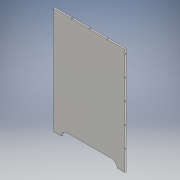
# Autodesk Inventor part: Venstre side mk2
Saved by Autodesk Inventor 2016 (Build 200138000, 138)
## iProperties
Created: 2015-10-17
Part Number: Venstre side mk2
Material: Generic
Document SubType Name: Modeling
Designer: iLyngklip
Density: 1 g/cm^3
Appearance: White
Author: iLyngklip
Autodesk Inventor part; units mm, degrees
ref_plane "YZ Plane" through (0, 0, 0) normal (1, 0, 0) x (0, 1, 0)
ref_plane "XZ Plane" through (0, 0, 0) normal (0, 1, 0) x (-1, 0, 0)
ref_plane "XY Plane" through (0, 0, 0) normal (0, 0, 1) x (1, 0, 0)
sketch "Sketch1" plane through (0, 0, 0) normal (0, 1, 0) x (-1, 0, 0)
  line L0 (160, 240) -> (-160, 240)
  line L1 (-160, 240) -> (-160, -240)
  line L2 (-160, -240) -> (160, -240)
  line L3 (160, -240) -> (160, 240)
  point P0 (0, 0)
  dimension "d0" = 320
  dimension "d1" = 480
  dimension "d2" = 240
  dimension "d3" = 160
  constraints: 8 end point, 2 parallel, 1 horizontal, 1 perpendicular
  measures "d0" distance of L1.end L2.end
  measures "d1" distance of L2.end L0.start
  measures "d2" distance from line of point (0, 0) L0
  measures "d3" distance from line of point (0, 0) L3
extrude "Tykkelse" add sketch "Sketch1" along normal blind 6
sketch "Sketch2" plane through (0, 6, 0) normal (0, 1, 0) x (1, 0, 0)
  line L0 (160, 240) -> (-160, 240) construction
  arc A0 (100, 215) -> (125, 240) centre (100, 240) ccw
  arc A1 (-125, 240) -> (-100, 215) centre (-100, 240) ccw
  line L1 (-100, 215) -> (100, 215)
  line L2 (-125, 240) -> (125, 240)
  point P0 (0, 0)
  dimension "d6" = 50
  dimension "d7" = 50
  dimension "d8" = 60
  dimension "d9" = 60
  constraints: 4 end point, 4 point on circle, 4 point on line, 2 centre point, 1 collinear, 1 horizontal, 1 tangent
  measures "d6" diameter of A0
  measures "d7" diameter of A1
  measures "d8" distance of L0.start A0.centre
  measures "d9" distance of A1.centre L0.end
extrude "Fødder" cut sketch "Sketch2" against normal up to surface (6 mm away)
sketch "Sketch7" plane through (0, 6, 0) normal (0, 1, 0) x (1, 0, 0)
  line L0 (-160, 146.5) -> (-153.679, 146.5) projected
  line L1 (-160, 149.5) -> (-160, 146.5) projected
  line L2 (-153.679, 149.5) -> (-160, 149.5) projected
  arc A0 (-152.2, 150.75) -> (-153.679, 149.5) centre (-152.2, 149.25) ccw projected
  line L3 (-150.8, 150.75) -> (-152.2, 150.75) projected
  arc A1 (-149.302, 149.3277) -> (-150.8, 150.75) centre (-150.8, 149.25) ccw projected
  arc A2 (-149.302, 146.6723) -> (-149.302, 149.3277) centre (-150, 148) ccw projected
  arc A3 (-150.8, 145.25) -> (-149.302, 146.6723) centre (-150.8, 146.75) ccw projected
  line L4 (-152.2, 145.25) -> (-150.8, 145.25) projected
  arc A4 (-153.679, 146.5) -> (-152.2, 145.25) centre (-152.2, 146.75) ccw projected
  line L5 (-150.8, 58.75) -> (-152.2, 58.75) projected
  arc A5 (-149.302, 57.3277) -> (-150.8, 58.75) centre (-150.8, 57.25) ccw projected
  arc A6 (-149.302, 54.6723) -> (-149.302, 57.3277) centre (-150, 56) ccw projected
  arc A7 (-150.8, 53.25) -> (-149.302, 54.6723) centre (-150.8, 54.75) ccw projected
  line L6 (-152.2, 53.25) -> (-150.8, 53.25) projected
  arc A8 (-153.679, 54.5) -> (-152.2, 53.25) centre (-152.2, 54.75) ccw projected
  line L7 (-160, 54.5) -> (-153.679, 54.5) projected
  line L8 (-160, 57.5) -> (-160, 54.5) projected
  line L9 (-153.679, 57.5) -> (-160, 57.5) projected
  arc A9 (-152.2, 58.75) -> (-153.679, 57.5) centre (-152.2, 57.25) ccw projected
  line L10 (-150.8, -33.25) -> (-152.2, -33.25) projected
  arc A10 (-149.302, -34.6723) -> (-150.8, -33.25) centre (-150.8, -34.75) ccw projected
  arc A11 (-149.302, -37.3277) -> (-149.302, -34.6723) centre (-150, -36) ccw projected
  arc A12 (-150.8, -38.75) -> (-149.302, -37.3277) centre (-150.8, -37.25) ccw projected
  line L11 (-152.2, -38.75) -> (-150.8, -38.75) projected
  arc A13 (-153.679, -37.5) -> (-152.2, -38.75) centre (-152.2, -37.25) ccw projected
  line L12 (-160, -37.5) -> (-153.679, -37.5) projected
  line L13 (-160, -34.5) -> (-160, -37.5) projected
  line L14 (-153.679, -34.5) -> (-160, -34.5) projected
  arc A14 (-152.2, -33.25) -> (-153.679, -34.5) centre (-152.2, -34.75) ccw projected
  arc A15 (-150.8, -130.75) -> (-149.302, -129.3277) centre (-150.8, -129.25) ccw projected
  line L15 (-152.2, -130.75) -> (-150.8, -130.75) projected
  arc A16 (-153.679, -129.5) -> (-152.2, -130.75) centre (-152.2, -129.25) ccw projected
  line L16 (-160, -129.5) -> (-153.679, -129.5) projected
  line L17 (-160, -126.5) -> (-160, -129.5) projected
  line L18 (-153.679, -126.5) -> (-160, -126.5) projected
  arc A17 (-152.2, -125.25) -> (-153.679, -126.5) centre (-152.2, -126.75) ccw projected
  line L19 (-150.8, -125.25) -> (-152.2, -125.25) projected
  arc A18 (-149.302, -126.6723) -> (-150.8, -125.25) centre (-150.8, -126.75) ccw projected
  arc A19 (-149.302, -129.3277) -> (-149.302, -126.6723) centre (-150, -128) ccw projected
  arc A20 (-149.302, -218.6723) -> (-150.8, -217.25) centre (-150.8, -218.75) ccw projected
  arc A21 (-149.302, -221.3277) -> (-149.302, -218.6723) centre (-150, -220) ccw projected
  arc A22 (-150.8, -222.75) -> (-149.302, -221.3277) centre (-150.8, -221.25) ccw projected
  line L20 (-152.2, -222.75) -> (-150.8, -222.75) projected
  arc A23 (-153.679, -221.5) -> (-152.2, -222.75) centre (-152.2, -221.25) ccw projected
  line L21 (-160, -221.5) -> (-153.679, -221.5) projected
  line L22 (-160, -218.5) -> (-160, -221.5) projected
  line L23 (-153.679, -218.5) -> (-160, -218.5) projected
  arc A24 (-152.2, -217.25) -> (-153.679, -218.5) centre (-152.2, -218.75) ccw projected
  line L24 (-150.8, -217.25) -> (-152.2, -217.25) projected
  line L25 (-81.5, -240) -> (-78.5, -240) projected
  line L26 (-81.5, -233.679) -> (-81.5, -240) projected
  arc A25 (-82.75, -232.2) -> (-81.5, -233.679) centre (-81.25, -232.2) ccw projected
  line L27 (-82.75, -230.8) -> (-82.75, -232.2) projected
  arc A26 (-81.3277, -229.302) -> (-82.75, -230.8) centre (-81.25, -230.8) ccw projected
  arc A27 (-78.6723, -229.302) -> (-81.3277, -229.302) centre (-80, -230) ccw projected
  arc A28 (-77.25, -230.8) -> (-78.6723, -229.302) centre (-78.75, -230.8) ccw projected
  line L28 (-77.25, -232.2) -> (-77.25, -230.8) projected
  arc A29 (-78.5, -233.679) -> (-77.25, -232.2) centre (-78.75, -232.2) ccw projected
  line L29 (-78.5, -240) -> (-78.5, -233.679) projected
  arc A30 (2.75, -230.8) -> (1.3277, -229.302) centre (1.25, -230.8) ccw projected
  line L30 (2.75, -232.2) -> (2.75, -230.8) projected
  arc A31 (1.5, -233.679) -> (2.75, -232.2) centre (1.25, -232.2) ccw projected
  line L31 (1.5, -240) -> (1.5, -233.679) projected
  line L32 (-1.5, -240) -> (1.5, -240) projected
  line L33 (-1.5, -233.679) -> (-1.5, -240) projected
  arc A32 (-2.75, -232.2) -> (-1.5, -233.679) centre (-1.25, -232.2) ccw projected
  line L34 (-2.75, -230.8) -> (-2.75, -232.2) projected
  arc A33 (-1.3277, -229.302) -> (-2.75, -230.8) centre (-1.25, -230.8) ccw projected
  arc A34 (1.3277, -229.302) -> (-1.3277, -229.302) centre (0, -230) ccw projected
  arc A35 (82.75, -230.8) -> (81.3277, -229.302) centre (81.25, -230.8) ccw projected
  line L35 (82.75, -232.2) -> (82.75, -230.8) projected
  arc A36 (81.5, -233.679) -> (82.75, -232.2) centre (81.25, -232.2) ccw projected
  line L36 (81.5, -240) -> (81.5, -233.679) projected
  line L37 (78.5, -240) -> (81.5, -240) projected
  line L38 (78.5, -233.679) -> (78.5, -240) projected
  arc A37 (77.25, -232.2) -> (78.5, -233.679) centre (78.75, -232.2) ccw projected
  line L39 (77.25, -230.8) -> (77.25, -232.2) projected
  arc A38 (78.6723, -229.302) -> (77.25, -230.8) centre (78.75, -230.8) ccw projected
  arc A39 (81.3277, -229.302) -> (78.6723, -229.302) centre (80, -230) ccw projected
  arc A40 (149.302, -218.6723) -> (149.302, -221.3277) centre (150, -220) ccw projected
  arc A41 (150.8, -217.25) -> (149.302, -218.6723) centre (150.8, -218.75) ccw projected
  line L40 (152.2, -217.25) -> (150.8, -217.25) projected
  arc A42 (153.679, -218.5) -> (152.2, -217.25) centre (152.2, -218.75) ccw projected
  line L41 (160, -218.5) -> (153.679, -218.5) projected
  line L42 (160, -221.5) -> (160, -218.5) projected
  line L43 (153.679, -221.5) -> (160, -221.5) projected
  arc A43 (152.2, -222.75) -> (153.679, -221.5) centre (152.2, -221.25) ccw projected
  line L44 (150.8, -222.75) -> (152.2, -222.75) projected
  arc A44 (149.302, -221.3277) -> (150.8, -222.75) centre (150.8, -221.25) ccw projected
  arc A45 (149.302, -126.6723) -> (149.302, -129.3277) centre (150, -128) ccw projected
  arc A46 (150.8, -125.25) -> (149.302, -126.6723) centre (150.8, -126.75) ccw projected
  line L45 (152.2, -125.25) -> (150.8, -125.25) projected
  arc A47 (153.679, -126.5) -> (152.2, -125.25) centre (152.2, -126.75) ccw projected
  line L46 (160, -126.5) -> (153.679, -126.5) projected
  line L47 (160, -129.5) -> (160, -126.5) projected
  line L48 (153.679, -129.5) -> (160, -129.5) projected
  arc A48 (152.2, -130.75) -> (153.679, -129.5) centre (152.2, -129.25) ccw projected
  line L49 (150.8, -130.75) -> (152.2, -130.75) projected
  arc A49 (149.302, -129.3277) -> (150.8, -130.75) centre (150.8, -129.25) ccw projected
  arc A50 (149.302, -34.6723) -> (149.302, -37.3277) centre (150, -36) ccw projected
  arc A51 (150.8, -33.25) -> (149.302, -34.6723) centre (150.8, -34.75) ccw projected
  line L50 (152.2, -33.25) -> (150.8, -33.25) projected
  arc A52 (153.679, -34.5) -> (152.2, -33.25) centre (152.2, -34.75) ccw projected
  line L51 (160, -34.5) -> (153.679, -34.5) projected
  line L52 (160, -37.5) -> (160, -34.5) projected
  line L53 (153.679, -37.5) -> (160, -37.5) projected
  arc A53 (152.2, -38.75) -> (153.679, -37.5) centre (152.2, -37.25) ccw projected
  line L54 (150.8, -38.75) -> (152.2, -38.75) projected
  arc A54 (149.302, -37.3277) -> (150.8, -38.75) centre (150.8, -37.25) ccw projected
  arc A55 (149.302, 57.3277) -> (149.302, 54.6723) centre (150, 56) ccw projected
  arc A56 (150.8, 58.75) -> (149.302, 57.3277) centre (150.8, 57.25) ccw projected
  line L55 (152.2, 58.75) -> (150.8, 58.75) projected
  arc A57 (153.679, 57.5) -> (152.2, 58.75) centre (152.2, 57.25) ccw projected
  line L56 (160, 57.5) -> (153.679, 57.5) projected
  line L57 (160, 54.5) -> (160, 57.5) projected
  line L58 (153.679, 54.5) -> (160, 54.5) projected
  arc A58 (152.2, 53.25) -> (153.679, 54.5) centre (152.2, 54.75) ccw projected
  line L59 (150.8, 53.25) -> (152.2, 53.25) projected
  arc A59 (149.302, 54.6723) -> (150.8, 53.25) centre (150.8, 54.75) ccw projected
  line L60 (160, 146.5) -> (160, 149.5) projected
  line L61 (153.679, 146.5) -> (160, 146.5) projected
  arc A60 (152.2, 145.25) -> (153.679, 146.5) centre (152.2, 146.75) ccw projected
  line L62 (150.8, 145.25) -> (152.2, 145.25) projected
  arc A61 (149.302, 146.6723) -> (150.8, 145.25) centre (150.8, 146.75) ccw projected
  arc A62 (149.302, 149.3277) -> (149.302, 146.6723) centre (150, 148) ccw projected
  arc A63 (150.8, 150.75) -> (149.302, 149.3277) centre (150.8, 149.25) ccw projected
  line L63 (152.2, 150.75) -> (150.8, 150.75) projected
  arc A64 (153.679, 149.5) -> (152.2, 150.75) centre (152.2, 149.25) ccw projected
  line L64 (160, 149.5) -> (153.679, 149.5) projected
  line L65 (160, 240) -> (125, 240) projected
  point P0 (0, 0)
  dimension "d224" = 92
  measures "d224" distance from line of L65 A62.centre
extrude "Monteringshuller" cut sketch "Sketch7" against normal blind 5
sketch "Sketch8" plane through (0, 6, 0) normal (0, 1, 0) x (1, 0, 0)
  circle A0 centre (122, -200) radius 8 projected
  circle A1 centre (-150, -200) radius 8 projected
  point P0 (0, 0)
extrude "Lejehuller" cut sketch "Sketch8" against normal blind 3.5
equation "\"d2\" = 0.5 * d1"
equation "\"d3\" = 0.5 * d0"
equation "\"d6\" = d7"
equation "\"d9\" = d8"
body "Solid1"
